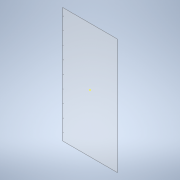
# Autodesk Inventor part: SP25V1 Acrilico
Saved by Autodesk Inventor 2021.2 (Build 252289000, 289)
## iProperties
Created: 2026-06-02
Part Number: SP25V1 Acrilico
Material: Cristal
Document SubType Name: Modeling
Designer: nelso
Density: 2.18 g/cm^3
Appearance: Transparente - Claro
Mass: 9370.9 g
Surface Area: 28808.3 cm^2
Volume: 4298.58 cm^3
Author: nelso
Autodesk Inventor part; units mm, degrees
ref_plane "YZ Plane" through (0, 0, 0) normal (1, 0, 0) x (0, 1, 0)
ref_plane "XZ Plane" through (0, 0, 0) normal (0, 1, 0) x (-1, 0, 0)
ref_plane "XY Plane" through (0, 0, 0) normal (0, 0, 1) x (1, 0, 0)
sketch "Sketch1" plane through (0, 0, 0) normal (0, 0, 1) x (1, 0, 0)
  line L0 (-390, -825) -> (390, -825)
  line L1 (390, -825) -> (390, 825)
  line L2 (390, 825) -> (-390, 825)
  line L3 (-390, 825) -> (-390, -825)
  line L4 (-390, -825) -> (390, 825) construction
  line L5 (390, -825) -> (-390, 825) construction
  point P0 (0, 0)
  dimension "d0" = 780
  dimension "d1" = 1650
  constraints: 12 end point, 2 midpoint, 2 parallel, 1 horizontal, 1 perpendicular
  measures "d0" distance of L2.end L1.end
  measures "d1" distance of L1.end L0.end
extrude "Extrusion1" add sketch "Sketch1" along normal blind 3
sketch "Sketch2" plane through (0, 0, 3) normal (0, 0, 1) x (1, 0, 0)
  point P0 (0, 0)
sketch "Sketch3" plane through (0, 0, 3) normal (0, 0, 1) x (1, 0, 0)
  line L0 (-390, 825) -> (-390, -825) projected
  line L1 (-390, 825) -> (-383.65, 825)
  line L2 (390, 825) -> (-390, 825) projected
  line L3 (-383.65, 825) -> (-383.65, -825)
  line L4 (-390, -825) -> (390, -825) projected
  line L5 (390, -825) -> (390, 825) projected
  line L6 (390, 825) -> (383.65, 825)
  line L7 (383.65, 825) -> (383.65, -825)
  circle A0 centre (-383.65, 720) radius 2.25
  circle A1 centre (-383.65, 540) radius 2.25
  circle A2 centre (-383.65, 360) radius 2.25
  circle A3 centre (-383.65, 180) radius 2.25
  circle A4 centre (-383.65, 0) radius 2.25
  circle A5 centre (-383.65, -180) radius 2.25
  circle A6 centre (-383.65, -360) radius 2.25
  circle A7 centre (-383.65, -540) radius 2.25
  circle A8 centre (-383.65, -720) radius 2.25
  circle A9 centre (453.25, 720) radius 2.25
  circle A10 centre (453.25, 540) radius 2.25
  circle A11 centre (453.25, 360) radius 2.25
  circle A12 centre (453.25, 180) radius 2.25
  circle A13 centre (453.25, 0) radius 2.25
  circle A14 centre (453.25, -180) radius 2.25
  circle A15 centre (453.25, -360) radius 2.25
  circle A16 centre (453.25, -540) radius 2.25
  circle A17 centre (453.25, -720) radius 2.25
  point P0 (0, 0)
  dimension "d6" = 6.35
  dimension "d7" = 6.35
  dimension "d9" = 4.5
  dimension "d12" = 180
  dimension "d15" = 836.9
  constraints: 18 centre point, 8 end point, 4 point on line, 2 perpendicular, 1 horizontal, 1 vertical, 34 other
  measures "d6" distance of L0.start L1.end
  measures "d7" distance of L2.start L6.end
  measures "d9" diameter of A0
  measures "d12" distance of A0.centre A1.centre
  measures "d15" distance of A0.centre A9.centre
extrude "Extrusion2" cut sketch "Sketch3" against normal up to surface (3 mm away) contours A0 L3 | L3 A0 | A8 L3 | L3 A8 | A1 L3 | L3 A1 | A7 L3 | L3 A7 | A2 L3 | L3 A2 | A6 L3 | L3 A6 | A3 L3 | L3 A3 | A5 L3 | L3 A5 | A4 L3 | L3 A4 | A9 | A10 | A11 | A12 | A13 | A14 | A15 | A16 | A17
body "Solid1"
